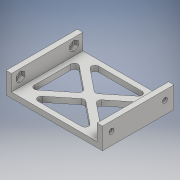
# Autodesk Inventor part: upper_leg_spacer
Saved by Autodesk Inventor 2018 (Build 220112000, 112)
## iProperties
Created: 2019-06-12
Part Number: upper_leg_spacer
Material: Generic
Document SubType Name: Modeling
Designer: Jasper
Density: 1 g/cm^3
Appearance: Default
Author: Jasper
Autodesk Inventor part; units mm, degrees
ref_plane "YZ Plane" through (0, 0, 0) normal (1, 0, 0) x (0, 1, 0)
ref_plane "XZ Plane" through (0, 0, 0) normal (0, 1, 0) x (-1, 0, 0)
ref_plane "XY Plane" through (0, 0, 0) normal (0, 0, 1) x (1, 0, 0)
sketch "Sketch1" plane through (0, 0, 0) normal (0, 0, 1) x (1, 0, 0)
  line L0 (-27, 20) -> (27, 20)
  line L1 (27, 20) -> (27, -20)
  line L2 (27, -20) -> (-27, -20)
  line L3 (-27, -20) -> (-27, 20)
  line L4 (-27, 20) -> (27, -20) construction
  line L5 (27, 20) -> (-27, -20) construction
  point P0 (0, 0)
  dimension "d0" = 54
  dimension "d1" = 40
  constraints: 12 end point, 2 midpoint, 2 parallel, 1 horizontal, 1 perpendicular
  measures "d0" distance of L1.end L2.end
  measures "d1" distance of L0.end L1.end
extrude "Extrusion1" add sketch "Sketch1" along normal blind 12
sketch "Sketch2" plane through (0, 0, 12) normal (0, 0, 1) x (1, 0, 0)
  line L0 (-24, -20) -> (24, -20)
  line L1 (24, -20) -> (24, 20)
  line L2 (24, 20) -> (-24, 20)
  line L3 (-24, 20) -> (-24, -20)
  line L4 (-24, -20) -> (24, 20) construction
  line L5 (24, -20) -> (-24, 20) construction
  point P0 (0, 0)
  dimension "d4" = 48
  dimension "d5" = 40
  constraints: 12 end point, 2 midpoint, 2 parallel, 1 horizontal, 1 perpendicular
  measures "d4" distance of L2.end L1.end
  measures "d5" distance of L1.end L0.end
extrude "Extrusion2" cut sketch "Sketch2" against normal blind 9
sketch "Sketch3" plane through (-24, -20, 12) normal (1, 0, 0) x (0, 0, -1)
  line L0 (9, 0) -> (0, 0) projected
  line L1 (0, 0) -> (0, 5)
  line L2 (0, 40) -> (0, 0) projected
  line L3 (0, 5) -> (0, 35)
  line L4 (0, 5) -> (4, 5)
  line L5 (0, 0) -> (0, 40) projected
  line L6 (0, 5) -> (4, 5) construction
  line L7 (0, 35) -> (4, 35)
  line L8 (0, 35) -> (4, 35) construction
  line L9 (1.2287, 35) -> (2.6144, 37.4)
  line L10 (2.6144, 37.4) -> (5.3856, 37.4)
  line L11 (5.3856, 37.4) -> (6.7713, 35)
  line L12 (6.7713, 35) -> (5.3856, 32.6)
  line L13 (5.3856, 32.6) -> (2.6144, 32.6)
  line L14 (2.6144, 32.6) -> (1.2287, 35)
  line L15 (1.2287, 5) -> (2.6144, 7.4)
  line L16 (2.6144, 7.4) -> (5.3856, 7.4)
  line L17 (5.3856, 7.4) -> (6.7713, 5)
  line L18 (6.7713, 5) -> (5.3856, 2.6)
  line L19 (5.3856, 2.6) -> (2.6144, 2.6)
  line L20 (2.6144, 2.6) -> (1.2287, 5)
  line L21 (9, 40) -> (9, 0) construction
  line L22 (9, 0) -> (9, 40) construction
  point P0 (12, 20)
  dimension "d8" = 5
  dimension "d9" = 30
  dimension "d10" = 180
  dimension "d11" = 4
  dimension "d12" = 0
  dimension "d13" = 4
  dimension "d14" = 0
  dimension "d15" = 4.8
  dimension "d16" = 4.8
  constraints: 36 end point, 3 collinear, 3 point on line, 2 coincident, 2 horizontal, 2 perpendicular, 26 other
  measures "d8" distance of L0.end L1.end
  measures "d9" distance of L1.end L3.end
  measures "d10" angle of L3 L1
  measures "d11" distance of L1.end L4.end
  measures "d12" distance between parallel lines of L4 L6
  measures "d13" distance of L3.end L7.end
  measures "d14" distance between parallel lines of L7 L8
  measures "d15" distance between parallel lines of L12 L9
  measures "d16" distance between parallel lines of L18 L15
extrude "Extrusion3" cut sketch "Sketch3" against normal blind 2
sketch "Sketch4" plane through (24, -20, 12) normal (-1, 0, 0) x (0, 0, 1)
  line L0 (-9, 0) -> (-9, 5)
  line L1 (-9, 40) -> (-9, 0) projected
  line L2 (-9, 5) -> (-9, 20)
  line L3 (-9, 20) -> (-1, 20)
  line L4 (-9, 5) -> (-5, 5)
  line L5 (-9, 5) -> (-5, 5) construction
  line L6 (-7.7713, 5) -> (-6.3856, 7.4)
  line L7 (-6.3856, 7.4) -> (-3.6144, 7.4)
  line L8 (-3.6144, 7.4) -> (-2.2287, 5)
  line L9 (-2.2287, 5) -> (-3.6144, 2.6)
  line L10 (-3.6144, 2.6) -> (-6.3856, 2.6)
  line L11 (-6.3856, 2.6) -> (-7.7713, 5)
  line L12 (-7.7713, 35) -> (-6.3856, 32.6)
  line L13 (-6.3856, 32.6) -> (-3.6144, 32.6)
  line L14 (-3.6144, 32.6) -> (-2.2287, 35)
  line L15 (-2.2287, 35) -> (-3.6144, 37.4)
  line L16 (-3.6144, 37.4) -> (-6.3856, 37.4)
  line L17 (-6.3856, 37.4) -> (-7.7713, 35)
  point P0 (-12, 20)
  dimension "d19" = 5
  dimension "d20" = 15
  dimension "d21" = 180
  dimension "d22" = 8
  dimension "d23" = 90
  dimension "d24" = 4
  dimension "d25" = 0
  dimension "d26" = 4.8
  constraints: 34 end point, 6 symmetric about line, 2 collinear, 2 horizontal, 2 point on line, 1 coincident, 1 perpendicular, 13 other
  measures "d19" distance of L0.start L0.end
  measures "d20" distance of L0.end L2.end
  measures "d21" angle of L2 L0
  measures "d22" distance of L2.end L3.end
  measures "d23" angle of L2 L3
  measures "d24" distance of L0.end L4.end
  measures "d25" distance between parallel lines of L4 L5
  measures "d26" distance between parallel lines of L9 L6
extrude "Extrusion4" cut sketch "Sketch4" against normal blind 2
sketch "Sketch6" plane through (24, -20, 12) normal (-1, 0, 0) x (0, 0, 1)
  line L0 (-9, 0) -> (-9, 5)
  line L1 (-9, 0) -> (-4, 0) construction
  line L2 (-9, 5) -> (-5, 5)
  line L3 (-9, 5) -> (-9, 20)
  line L4 (-9, 5) -> (6, 5) construction
  line L5 (-9, 20) -> (-1, 20)
  circle A0 centre (-5, 5) radius 1.35
  circle A1 centre (-5, 35) radius 1.35
  point P0 (-12, 20)
  dimension "d29" = 5
  dimension "d30" = 90
  dimension "d31" = 4
  dimension "d32" = 90
  dimension "d33" = 15
  dimension "d34" = 90
  dimension "d35" = 8
  dimension "d36" = 90
  dimension "d37" = 2.7
  constraints: 12 end point, 4 perpendicular, 2 centre point, 2 horizontal, 2 vertical, 1 coincident, 1 symmetric about line, 1 other
  measures "d29" distance of L0.start L0.end
  measures "d30" angle of L1 L0
  measures "d31" distance of L0.end L2.end
  measures "d32" angle of L0 L2
  measures "d33" distance of L0.end L3.end
  measures "d34" angle of L4 L3
  measures "d35" distance of L3.end L5.end
  measures "d36" angle of L3 L5
  measures "d37" diameter of A0
extrude "Extrusion5" cut sketch "Sketch6" against normal up to surface (3 mm away)
sketch "Sketch7" plane through (-27, -20, 0) normal (-1, 0, 0) x (0, 0, 1)
  line L0 (12, 0) -> (12, 40) projected
  line L1 (12, 0) -> (12, 5)
  line L2 (12, 0) -> (17, 0) construction
  line L3 (12, 5) -> (8, 5)
  line L4 (12, 5) -> (12, 20)
  line L5 (12, 5) -> (27, 5) construction
  line L6 (12, 20) -> (0, 20)
  circle A0 centre (8, 5) radius 1.35
  circle A1 centre (8, 35) radius 1.35
  dimension "d40" = 5
  dimension "d41" = 90
  dimension "d42" = 4
  dimension "d43" = 90
  dimension "d44" = 15
  dimension "d45" = 90
  dimension "d46" = 2.7
  constraints: 12 end point, 3 perpendicular, 2 centre point, 2 collinear, 2 horizontal, 1 coincident, 1 symmetric about line, 1 other
  measures "d40" distance of L0.start L1.end
  measures "d41" angle of L2 L1
  measures "d42" distance of L1.end L3.end
  measures "d43" angle of L3 L1
  measures "d44" distance of L1.end L4.end
  measures "d45" angle of L5 L4
  measures "d46" diameter of A0
extrude "Extrusion6" cut sketch "Sketch7" against normal up to surface (3 mm away)
sketch "Sketch8" plane through (0, 0, 3) normal (0, 0, 1) x (1, 0, 0)
  line L0 (24, -20) -> (-24, -20) projected
  line L1 (-24, -20) -> (-21, -20)
  line L2 (-24, -20) -> (-21, -20) construction
  line L3 (-24, 20) -> (24, 20) projected
  line L4 (-21, -20) -> (-21, -17)
  line L5 (-21, -20) -> (-18, -20) construction
  line L6 (-21, -17) -> (21, -17) construction
  line L7 (21, -17) -> (21, 17) construction
  line L8 (21, 17) -> (-21, 17)
  line L9 (-21, 17) -> (-21, -17)
  line L10 (21, -17) -> (21, -15)
  line L11 (21, -17) -> (23, -17) construction
  line L12 (21, -17) -> (19, -17)
  line L13 (21, -17) -> (23, -17) construction
  line L14 (21, -15) -> (41, -15) construction
  line L15 (-21, 17) -> (-21, 15)
  line L16 (21, 17) -> (-21, -17)
  line L17 (-21, 17) -> (21, -17)
  line L18 (-19.7416, -18.5545) -> (22.2584, 15.4455) construction
  line L19 (22.2584, 15.4455) -> (19.7416, 18.5545)
  line L20 (19.7416, 18.5545) -> (-22.2584, -15.4455) construction
  line L21 (-22.2584, -15.4455) -> (-19.7416, -18.5545)
  line L22 (-19.7416, -18.5545) -> (19.7416, 18.5545) construction
  line L23 (22.2584, 15.4455) -> (-22.2584, -15.4455) construction
  line L24 (-22.2584, 15.4455) -> (19.7416, -18.5545) construction
  line L25 (19.7416, -18.5545) -> (22.2584, -15.4455)
  line L26 (22.2584, -15.4455) -> (-19.7416, 18.5545) construction
  line L27 (-19.7416, 18.5545) -> (-22.2584, 15.4455)
  line L28 (-22.2584, 15.4455) -> (22.2584, -15.4455) construction
  line L29 (19.7416, -18.5545) -> (-19.7416, 18.5545) construction
  line L30 (0, -2.5732) -> (-17.8214, -17)
  line L31 (0, -2.5732) -> (17.8214, -17)
  line L32 (17.8214, -17) -> (-17.8214, -17)
  line L33 (24, -20) -> (-24, -20) construction
  line L34 (24, 20) -> (24, -20) construction
  line L35 (-24, 20) -> (24, 20) construction
  line L36 (-24, -20) -> (-24, 20) construction
  line L37 (-21, 0) -> (21, 0) construction
  line L38 (0, 17) -> (0, -17) construction
  line L39 (0, 2.5732) -> (-17.8214, 17)
  line L40 (0, 2.5732) -> (17.8214, 17)
  line L41 (17.8214, 17) -> (-17.8214, 17)
  line L42 (3.1786, 0) -> (21, -14.4268)
  line L43 (3.1786, 0) -> (21, 14.4268)
  line L44 (21, 14.4268) -> (21, -14.4268)
  line L45 (-3.1786, 0) -> (-21, -14.4268)
  line L46 (-3.1786, 0) -> (-21, 14.4268)
  line L47 (-21, 14.4268) -> (-21, -14.4268)
  point P0 (0, 0)
  dimension "d49" = 3
  dimension "d50" = 0
  dimension "d52" = 3
  dimension "d53" = 90
  dimension "d54" = 42
  dimension "d55" = 34
  dimension "d56" = 2
  dimension "d57" = 90
  dimension "d58" = 2
  dimension "d59" = 180
  dimension "d64" = 2
  dimension "d65" = 4
  dimension "d66" = 54.037
  dimension "d67" = 4
  dimension "d68" = 54.037
  constraints: 84 end point, 12 point on line, 9 parallel, 8 midpoint, 6 horizontal, 6 symmetric about line, 5 collinear, 4 equal length, 4 perpendicular
  measures "d49" distance of L0.end L1.end
  measures "d50" distance between parallel lines of L1 L2
  measures "d52" distance of L2.end L4.end
  measures "d53" angle of L5 L4
  measures "d54" distance of L8.end L7.end
  measures "d55" distance of L7.end L6.end
  measures "d56" distance of L6.end L10.end
  measures "d57" angle of L11 L10
  measures "d58" distance of L6.end L12.end
  measures "d59" angle of L12 L13
  measures "d64" distance of L8.end L15.end
  measures "d65" distance of L19.end L18.end
  measures "d66" distance of L19.end L20.end
  measures "d67" distance of L25.end L24.end
  measures "d68" distance of L25.end L26.end
extrude "Extrusion7" cut sketch "Sketch8" against normal up to surface (3 mm away) contours L40 L39 L8 | L9 L46 L45 | L31 L32 L30 | L43 L44 L42
fillet "Fillet1" radius 2 12 edges at (-17.8214, -17, 1.5) (-21, -14.4268, 1.5) (-21, 14.4268, 1.5) (-17.8214, 17, 1.5) (21, 14.4268, 1.5) (17.8214, 17, 1.5) (0, 2.5732, 1.5) (-3.1786, 0, 1.5) (3.1786, 0, 1.5) (0, -2.5732, 1.5) (21, -14.4268, 1.5) (17.8214, -17, 1.5)
body "Solid1"
